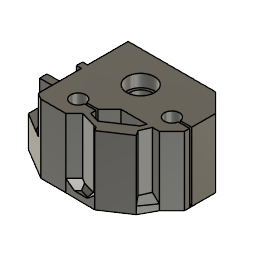
rolls mount right (Autodesk Fusion 360 design; units mm, degrees)
Autodesk Fusion 360 part; units mm, degrees
sketch "Szkic1" plane through (0, 0, 0) normal (0, 0, 1) x (1, 0, 0)
  line L0 (25, -25) -> (25, 25)
  line L1 (35, -10.8) -> (50, -10.8)
  line L2 (35, -9.2) -> (50, -9.2)
  line L3 (-30, -50) -> (0, -50)
  line L4 (0, 0) -> (0, 25)
  line L5 (22, 22) -> (-22, -22) construction
  line L6 (-35.000001, 12.5) -> (-40.000001, 12.5)
  line L7 (-40.000001, 17.5) -> (-40.000001, 12.5)
  line L8 (-30, -25) -> (-30, -50)
  line L9 (-55.000001, 5) -> (-55.000001, -35.000001)
  circle A0 centre (35, -10) radius 6
  line L10 (-25, 25) -> (-35, 25)
  line L11 (-35, 5) -> (-35, 25)
  circle A1 centre (-45, 15) radius 3
  line L12 (-25, 25) -> (-25, -25)
  line L13 (-15, -35.8) -> (0, -35.8)
  line L14 (-15, -34.2) -> (0, -34.2)
  line L15 (-15.5, -15.5) -> (15.5, 15.5) construction
  line L16 (-55, 25) -> (-55.000001, 5)
  line L17 (25, -25) -> (50, -25)
  line L18 (50, -25) -> (50, 5)
  line L19 (-25, -25) -> (-30, -25)
  line L20 (-35, 5) -> (-55.000001, 5)
  line L21 (50, 5) -> (22, 5)
  line L22 (-22, 22) -> (22, -22) construction
  line L23 (-25, -25) -> (25, -25)
  circle A2 centre (-15, -35) radius 6
  line L24 (-35.000001, 17.5) -> (-40.000001, 17.5)
  line L25 (-55.000001, -35.000001) -> (-30, -35.000001)
  line L26 (15.5, -15.5) -> (-14.262563, 14.262563) construction
  line L27 (0, -50) -> (0, -25)
  line L28 (-35, 25) -> (-55, 25)
  line L29 (25, 25) -> (-25, 25)
  circle A3 centre (0, 0) radius 11.5
  line L30 (-55, 25) -> (-55, 60)
  line L31 (-55, 60) -> (-35, 60)
  line L32 (-35, 60) -> (-35, 25)
  circle A4 centre (-45, 45) radius 3
  line L33 (50, 5) -> (25, 25)
  line L34 (-30, -50) -> (-55.000001, -35.000001)
  line L35 (-25, 25) -> (-25, 60)
  line L36 (-25, 60) -> (-35, 60)
  dimension "d2" = 12
  dimension "d3" = 12
  dimension "d6" = 25
  dimension "d11" = 6
  dimension "d12" = 23
  dimension "d13" = 6
  constraint coincident L4.start L5
  constraint coincident L4.start L22
  constraint perpendicular L0 L17
  constraint perpendicular L12 L19
  constraint perpendicular L8 L19
  constraint perpendicular L3 L8
  constraint midpoint L27.end L23
  constraint perpendicular L23 L27
  constraint coincident L4.start A3.centre
  constraint vertical L4
  constraint vertical L11
  constraint coincident L4.start L15
  constraint coincident L4.start L26
  constraint coincident L15.start L5
  constraint vertical L7
  constraint perpendicular L7 L24
  constraint perpendicular L6 L7
  constraint perpendicular L11 L20
  constraint perpendicular L9 L20
  constraint perpendicular L8 L25
  constraint perpendicular L11 L28
  constraint perpendicular L28 L30
  constraint perpendicular L30 L31
  constraint perpendicular L28 L32
  constraint perpendicular L10 L35
  constraint perpendicular L32 L36
  measures "d2" diameter of A2
  measures "d3" diameter of A0
  measures "d6" distance of L4.start L4.end
  measures "d11" diameter of A1
  measures "d12" diameter of A3
  measures "d13" diameter of A4
extrude "Wyciągnięcie proste1" add sketch "Szkic1" along normal blind 10 contours L0 L12 L23 L29 | L0 L1 L2 A0 L17 L18 L21 | L0 L21 L33 | L3 L8 L13 L14 L19 L23 A2 L27 | L8 L9 L10 L11 L12 L19 L20 L25 | L10 L32 L35 L36 | L8 L25 L34 | L6 L7 L11 L24 picked at (-20.495383, -0.188093) picked at (36.89922, -21.986434) picked at (33.333334, 11.666667) picked at (-15.06036, -46.999089) picked at (-46.666667, -18.333334) picked at (-28.333333, 48.333333) picked at (-38.333334, -40) picked at (-38.333334, 15.833334) makes body 1
extrude "Wyciągnięcie proste2" add sketch "Szkic1" against normal blind 10 separate body contours L6 L7 L11 L16 L20 L24 L28 | L28 L30 L31 L32 | L6 L7 L11 L24 picked at (-45.07473, 7.33613) picked at (-44.92527, 30.669463) picked at (-38.333334, 15.833334) makes body 2
extrude "Wyciągnięcie proste3" add sketch "Szkic1" against normal blind 15 contours L0 L12 L23 L29 | L0 L1 L2 A0 L17 L18 L21 | L0 L21 L33 | L3 L8 L13 L14 L19 L23 A2 L27 | L8 L9 L10 L11 L12 L19 L20 L25 | L10 L32 L35 L36 | L8 L25 L34 picked at (-20.495383, -0.188093) picked at (36.89922, -21.986434) picked at (33.333334, 11.666667) picked at (-15.06036, -46.999089) picked at (-46.666667, -18.333334) picked at (-28.333333, 48.333333) picked at (-38.333334, -40) bodies 1 2
sketch "Szkic2" plane through (0, 0, -15) normal (0, 0, -1) x (1, 0, 0)
  circle A0 centre (0, 0) radius 11.5
  line L0 (50, 9.2) -> (40.946428, 9.2)
  arc A1 (40.946427, 10.8) -> (40.946428, 9.2) centre (35, 10) ccw
  line L1 (40.946427, 10.8) -> (50, 10.8)
  line L2 (50, 10.8) -> (50, 25)
  line L3 (50, 25) -> (0, 25)
  line L4 (0, 25) -> (0, 34.2)
  line L5 (0, 34.2) -> (-9.053573, 34.2)
  arc A2 (-9.053573, 35.8) -> (-9.053573, 34.2) centre (-15, 35) ccw
  line L6 (-9.053573, 35.8) -> (0, 35.8)
  line L7 (0, 35.8) -> (0, 50)
  line L8 (0, 50) -> (-30, 50)
  line L9 (-30, 50) -> (-55.000001, 35.000001)
  line L10 (-55.000001, 35.000001) -> (-55.000001, -5)
  line L11 (-55.000001, -5) -> (-35, -5)
  line L12 (-35, -5) -> (-35, -60)
  line L13 (-35, -60) -> (-25, -60)
  line L14 (-25, -60) -> (-25, -25)
  line L15 (-25, -25) -> (25, -25)
  line L16 (25, -25) -> (50, -5)
  line L17 (50, -5) -> (50, 9.2)
  circle A3 centre (0, 0) radius 9
  dimension "d20" = 18
  constraint coincident A0.centre A3.centre
  measures "d20" diameter of A3
extrude "Wyciągnięcie proste4" add sketch "Szkic2" against normal blind 15 contours A0 picked at (10.590344, -1.018455) bodies 1
chamfer "Fazowanie1" distance 9.2 angle 45 1 edges at (0, -25, -2.5) on bodies 1
chamfer "Fazowanie2" distance 10 angle 45 1 edges at (0, -50, -2.5) on bodies 1
chamfer "Fazowanie3" distance 10 angle 45 1 edges at (50, -25, -2.5) on bodies 1
chamfer "Fazowanie4" distance 15 angle 45 1 edges at (-25, 25, -2.5) on bodies 1
sketch "Szkic3" plane through (0, 0, 10) normal (0, 0, 1) x (-1, 0, 0)
  line L0 (-40, 25) -> (-50, 15)
  line L1 (-50, 15) -> (-50, 10.8)
  line L2 (-50, 10.8) -> (-40.946427, 10.8)
  arc A0 (-40.946428, 9.2) -> (-40.946427, 10.8) centre (-35, 10) ccw
  line L3 (-40.946428, 9.2) -> (-50, 9.2)
  line L4 (-50, 9.2) -> (-50, -5)
  line L5 (-50, -5) -> (-25, -25)
  line L6 (-25, -25) -> (10, -25)
  line L7 (10, -25) -> (25, -40)
  line L8 (25, -40) -> (25, -60)
  line L9 (25, -60) -> (35, -60)
  line L10 (35, -60) -> (35.000001, -17.5)
  line L11 (35.000001, -17.5) -> (40.000001, -17.5)
  line L12 (40.000001, -17.5) -> (40.000001, -12.5)
  line L13 (40.000001, -12.5) -> (35, -12.5)
  line L14 (35, -12.5) -> (35, -5)
  line L15 (35, -5) -> (55.000001, -5)
  line L16 (55.000001, -5) -> (55.000001, 35.000001)
  line L17 (55.000001, 35.000001) -> (30, 50)
  line L18 (30, 50) -> (10, 50)
  line L19 (10, 50) -> (0, 40)
  line L20 (0, 40) -> (0, 35.8)
  line L21 (0, 35.8) -> (9.053573, 35.8)
  arc A1 (9.053573, 34.2) -> (9.053573, 35.8) centre (15, 35) ccw
  line L22 (9.053573, 34.2) -> (0, 34.2)
  line L23 (0, 34.2) -> (-9.2, 25)
  line L24 (-9.2, 25) -> (-40, 25)
  circle A2 centre (0, 0) radius 11.5
  line L25 (55.000001, -5) -> (35, -5)
  line L26 (35, -5) -> (35, 5)
  line L27 (35, 5) -> (55.000001, 5)
  line L28 (55.000001, 5) -> (55.000001, -5)
  constraint perpendicular L25 L26
  constraint parallel L25 L27
  constraint parallel L26 L28
  constraint coincident L14.end L15.start
  constraint perpendicular L14 L25
extrude "Wyciągnięcie proste5" add sketch "Szkic3" along normal blind 25 contours L15 L16 L25 L26 L27 L28 picked at (41.666667, 1.666667) bodies 1
sketch "Szkic4" plane through (0, -5, 0) normal (0, -1, 0) x (1, 0, 0)
  line L0 (-55.000001, 10) -> (-35, 10)
  line L1 (-35, 10) -> (-35, 35)
  line L2 (-35, 35) -> (-55.000001, 35)
  line L3 (-55.000001, 35) -> (-55.000001, 10)
  circle A0 centre (-45, 25) radius 3
  dimension "d29" = 6
  measures "d29" diameter of A0
extrude "Wyciągnięcie proste6" cut sketch "Szkic4" against normal blind 32 contours A0 picked at (-45.440071, 26.928078) bodies 1
chamfer "Fazowanie5" distance 5 angle 45 1 edges at (-45, -5, 10) on bodies 1
sketch "Szkic5" plane through (0, -5, 0) normal (0, -1, 0) x (1, 0, 0)
  line L0 (-55.000001, 15) -> (-35, 15)
  line L1 (-35, 15) -> (-35, 35)
  line L2 (-35, 35) -> (-55.000001, 35)
  line L3 (-55.000001, 35) -> (-55.000001, 15)
  circle A0 centre (-45, 25) radius 3
  line L4 (-46.500001, 28) -> (-43.500001, 28)
  line L5 (-43.500001, 28) -> (-43.500001, 26)
  line L6 (-46.500001, 28) -> (-46.500001, 27.795438)
  line L7 (-46.500001, 27.795438) -> (-46.500001, 26)
  constraint horizontal L4
  constraint perpendicular L4 L5
  constraint perpendicular L4 L6
  constraint parallel L6 L7
extrude "Wyciągnięcie proste7" cut sketch "Szkic5" against normal blind 23 contours A0 L4 L5 | A0 L4 L6 L7 picked at (-43.617317, 27.789905) picked at (-46.141503, 27.889805) bodies 1
sketch "Szkic6" plane through (0, 0, -15) normal (0, 0, -1) x (1, 0, 0)
  circle A0 centre (0, 0) radius 9
  line L0 (50, 15) -> (40, 25)
  line L1 (40, 25) -> (9.2, 25)
  line L2 (9.2, 25) -> (0, 34.2)
  line L3 (0, 34.2) -> (-9.053573, 34.2)
  arc A1 (-9.053573, 35.8) -> (-9.053573, 34.2) centre (-15, 35) ccw
  line L4 (-9.053573, 35.8) -> (0, 35.8)
  line L5 (0, 35.8) -> (0, 40)
  line L6 (0, 40) -> (-10, 50)
  line L7 (-10, 50) -> (-30, 50)
  line L8 (-30, 50) -> (-55.000001, 35.000001)
  line L9 (-55.000001, 35.000001) -> (-55.000001, -5)
  line L10 (-55.000001, -5) -> (-35, -5)
  line L11 (-35, -5) -> (-35, -60)
  line L12 (-35, -60) -> (-25, -60)
  line L13 (-25, -60) -> (-25, -40)
  line L14 (-25, -40) -> (-10, -25)
  line L15 (-10, -25) -> (25, -25)
  line L16 (25, -25) -> (50, -5)
  line L17 (50, -5) -> (50, 9.2)
  line L18 (50, 9.2) -> (40.946428, 9.2)
  arc A2 (40.946427, 10.8) -> (40.946428, 9.2) centre (35, 10) ccw
  line L19 (40.946427, 10.8) -> (50, 10.8)
  line L20 (50, 10.8) -> (50, 15)
  line L21 (50, 9.2) -> (40.946428, 9.2)
  line L22 (40.946428, 9.2) -> (40.946427, 10.8)
  line L23 (40.946427, 10.8) -> (50, 10.8)
  line L24 (50, 10.8) -> (50, 9.2)
  line L25 (0, 35.8) -> (-9.053573, 35.8)
  line L26 (-9.053573, 35.8) -> (-9.053573, 34.2)
  line L27 (-9.053573, 34.2) -> (0, 34.2)
  line L28 (0, 34.2) -> (0, 35.8)
  constraint perpendicular L21 L22
  constraint parallel L21 L23
  constraint parallel L22 L24
  constraint parallel L18 L21
  constraint coincident L17.end L18.start
  constraint perpendicular L25 L26
  constraint parallel L25 L27
  constraint parallel L26 L28
  constraint perpendicular L5 L25
  constraint coincident L4.end L5.start
extrude "Wyciągnięcie proste8" add sketch "Szkic6" against normal blind 1 contours L18 L19 L21 L22 L23 L24 | L3 L4 L25 L26 L27 L28 picked at (46.982142, 10.266667) picked at (-3.017858, 34.733333) bodies 1
sketch "Szkic7" plane through (0, 0, -10) normal (0, 0, -1) x (1, 0, 0)
  circle A0 centre (-45, -45) radius 3
  circle A1 centre (-45, -15) radius 3
  line L0 (-55.000001, -5) -> (-55, -25)
  line L1 (-55, -25) -> (-55, -60)
  line L2 (-55, -60) -> (-35, -60)
  line L3 (-35, -60) -> (-35, -5)
  line L4 (-35, -5) -> (-55.000001, -5)
  circle A2 centre (-45, -15) radius 5.5
  circle A3 centre (-45, -45) radius 5.5
  dimension "d37" = 11
  dimension "d38" = 11
  constraint concentric A1 A2
  constraint concentric A0 A3
  measures "d37" diameter of A2
  measures "d38" diameter of A3
extrude "Wyciągnięcie proste9" add sketch "Szkic7" along normal blind 5 contours L0 L1 L2 L3 L4 picked at (-45.137005, -56.828207) bodies 1
extrude "Wyciągnięcie proste10" add sketch "Szkic7" along normal blind 0.2 contours A0 | A1 | A2 | A3 picked at (-45.57473, -43.136771) picked at (-44.709389, -13.071922) picked at (-40.364979, -15.422286) picked at (-40.35381, -45.273244) bodies 1
sketch "Szkic8" plane through (0, 0, 0) normal (0, 0, 1) x (1, 0, 0)
  circle A0 centre (0, 0) radius 11.1
  circle A1 centre (0, 0) radius 11.5
  dimension "d43" = 22.2
  dimension "d44" = 23
  constraint coincident A0.centre A1.centre
  constraint concentric A0 A1
  measures "d43" diameter of A0
  measures "d44" diameter of A1
extrude "Wyciągnięcie proste11" add sketch "Szkic8" along normal blind 10 contours A1 picked at (11.282526, -1.122785) bodies 1
extrude "Wyciągnięcie proste12" cut 1 faces at (-45.222521, 5, 10.691739) along direction (0, -1, 0) blind 25 on bodies 1 bodies 1
extrude "Wyciągnięcie proste13" cut 1 faces at (-40.000001, 15.833334, 3.333333) along direction (1, 0, 0) blind 5 on bodies 1 bodies 1
sketch "Szkic9" plane through (0, 0, 0) normal (0, 0, 1) x (-1, 0, 0)
  line L0 (35, 20) -> (35, -60)
  line L1 (35, -60) -> (55, -60)
  line L2 (55, -60) -> (55, -25)
  line L3 (55, -25) -> (55.000001, -5)
  line L4 (55.000001, -5) -> (55.000001, 20)
  line L5 (55.000001, 20) -> (35, 20)
  circle A0 centre (45, -45) radius 3
  circle A1 centre (45, -15) radius 3
  circle A2 centre (45.000001, 10) radius 3
  line L6 (35.000001, 7.5) -> (35.000001, 12.5)
  line L7 (35.000001, 12.5) -> (39.000001, 12.5)
  line L8 (39.000001, 12.5) -> (39.000001, 7.5)
  line L9 (39.000001, 7.5) -> (35.000001, 7.5)
  dimension "d51" = 6
  dimension "d52" = 4
  constraint perpendicular L6 L7
  constraint parallel L6 L8
  constraint parallel L7 L9
  measures "d51" diameter of A2
extrude "Wyciągnięcie proste14" add sketch "Szkic9" along normal blind 10 contours L0 L6 L7 L8 L9 picked at (37.666667, 9.166667) bodies 1
extrude "Wyciągnięcie proste15" cut sketch "Szkic9" against normal blind 31 contours A2 picked at (44.425271, 11.863229) bodies 1
sketch "Szkic10" plane through (0, 0, 10) normal (0, 0, 1) x (-1, 0, 0)
  line L0 (35, -60) -> (35.000001, 7.5)
  line L1 (35.000001, 7.5) -> (39.000001, 7.5)
  line L2 (39.000001, 7.5) -> (39.000001, 12.5)
  line L3 (39.000001, 12.5) -> (35.000001, 12.5)
  line L4 (35.000001, 12.5) -> (35, 20)
  line L5 (35, 20) -> (55.000001, 20)
  line L6 (55.000001, 20) -> (55.000001, 35.000001)
  line L7 (55.000001, 35.000001) -> (30, 50)
  line L8 (30, 50) -> (10, 50)
  line L9 (10, 50) -> (0, 40)
  line L10 (0, 40) -> (0, 35.8)
  line L11 (0, 35.8) -> (9.053573, 35.8)
  arc A0 (9.053573, 34.2) -> (9.053573, 35.8) centre (15, 35) ccw
  line L12 (9.053573, 34.2) -> (0, 34.2)
  line L13 (0, 34.2) -> (-9.2, 25)
  line L14 (-9.2, 25) -> (-40, 25)
  line L15 (-40, 25) -> (-50, 15)
  line L16 (-50, 15) -> (-50, 10.8)
  line L17 (-50, 10.8) -> (-40.946427, 10.8)
  arc A1 (-40.946428, 9.2) -> (-40.946427, 10.8) centre (-35, 10) ccw
  line L18 (-40.946428, 9.2) -> (-50, 9.2)
  line L19 (-50, 9.2) -> (-50, -5)
  line L20 (-50, -5) -> (-25, -25)
  line L21 (-25, -25) -> (10, -25)
  line L22 (10, -25) -> (25, -40)
  line L23 (25, -40) -> (25, -60)
  line L24 (25, -60) -> (35, -60)
  circle A2 centre (0, 0) radius 11.1
  line L25 (55.000001, 20) -> (35, 20)
  line L26 (35, 20) -> (35, 26)
  line L27 (35, 26) -> (55.000001, 26)
  line L28 (55.000001, 26) -> (55.000001, 20)
  dimension "d57" = 6
  constraint perpendicular L25 L26
  constraint parallel L25 L27
  constraint parallel L26 L28
  constraint coincident L4.end L5.start
  constraint parallel L5 L25
extrude "Wyciągnięcie proste16" add sketch "Szkic10" along normal blind 20 contours L5 L6 L25 L26 L27 L28 picked at (41.666667, 24) bodies 1
sketch "Szkic11" plane through (0, -26, 0) normal (0, -1, 0) x (1, 0, 0)
  line L0 (-55.000001, 10) -> (-35, 10)
  line L1 (-35, 10) -> (-35, 30)
  line L2 (-35, 30) -> (-55.000001, 30)
  line L3 (-55.000001, 30) -> (-55.000001, 10)
  circle A0 centre (-45.000001, 20) radius 3
  dimension "d60" = 6
  measures "d60" diameter of A0
extrude "Wyciągnięcie proste17" cut sketch "Szkic11" against normal blind 26 contours A0 picked at (-45.440072, 21.928078) bodies 1
chamfer "Fazowanie6" distance 20 angle 45 1 edges at (-35, -23, 10) on bodies 1
chamfer "Fazowanie7" distance 3 angle 45 1 edges at (-35, -26, 10) on bodies 1
sketch "Szkic12" plane through (0, 0, -15) normal (0, 0, -1) x (1, 0, 0)
  circle A0 centre (-45.000001, 10) radius 3
  circle A1 centre (-45, -15) radius 5.5
  circle A2 centre (-45, -45) radius 5.5
  arc A3 (40.946427, 10.8) -> (40.946428, 9.2) centre (35, 10) ccw
  line L0 (40.946427, 10.8) -> (40.946428, 9.2)
  line L1 (50, 9.2) -> (50, 10.8)
  line L2 (50, 10.8) -> (50, 15)
  line L3 (50, 15) -> (40, 25)
  line L4 (40, 25) -> (9.2, 25)
  line L5 (9.2, 25) -> (0, 34.2)
  line L6 (0, 34.2) -> (0, 40)
  line L7 (0, 40) -> (-10, 50)
  line L8 (-10, 50) -> (-30, 50)
  line L9 (-30, 50) -> (-55.000001, 35.000001)
  line L10 (-55.000001, 35.000001) -> (-55.000001, -5)
  line L11 (-55.000001, -5) -> (-55, -25)
  line L12 (-55, -25) -> (-55, -60)
  line L13 (-55, -60) -> (-25, -60)
  line L14 (-25, -60) -> (-25, -40)
  line L15 (-25, -40) -> (-10, -25)
  line L16 (-10, -25) -> (25, -25)
  line L17 (25, -25) -> (50, -5)
  line L18 (50, -5) -> (50, 9.2)
  circle A4 centre (0, 0) radius 9
  line L19 (-9.053573, 35.8) -> (-9.053573, 34.2)
  arc A5 (-9.053573, 35.8) -> (-9.053573, 34.2) centre (-15, 35) ccw
  circle A6 centre (-45.000001, 10) radius 5.5
  dimension "d65" = 11
  constraint concentric A0 A6
  measures "d65" diameter of A6
extrude "Wyciągnięcie proste18" cut sketch "Szkic12" against normal blind 5 contours A6 picked at (-40.36498, 9.577714) bodies 1
extrude "Wyciągnięcie proste19" cut 1 faces at (-45.669792, 43.839886, -10.2) along direction (0, 0, 1) blind 0.2 on bodies 1 bodies 1
extrude "Wyciągnięcie proste20" cut 1 faces at (-43.619823, 11.993504, -10.2) along direction (0, 0, 1) blind 0.2 on bodies 1 bodies 1
extrude "Wyciągnięcie proste21" cut 3 faces at (-40.36498, -9.577714, -10) (-40.364979, 15.422286, -10) (-40.364979, 45.422286, -10) along direction (0, 0, 1) blind 4 on bodies 1 bodies 1
sketch "Szkic13" plane through (0, 0, -6) normal (0, 0, -1) x (1, 0, 0)
  circle A0 centre (-45, -45) radius 3
  circle A1 centre (-45, -45) radius 5.5
  circle A2 centre (-45, -15) radius 5.5
  circle A3 centre (-45, -15) radius 5.5
  circle A4 centre (-45, -45) radius 5.5
  circle A5 centre (-45.000001, 10) radius 5.5
  dimension "d75" = 11
  dimension "d76" = 11
  dimension "d77" = 11
  constraint concentric A2 A3
  constraint concentric A0 A4
  measures "d75" diameter of A2
  measures "d76" diameter of A4
  measures "d77" diameter of A5
extrude "Wyciągnięcie proste22" add sketch "Szkic13" 1 faces at (-40.364979, 45.422286, -6) along normal blind 0.2 contours A0 | A2 A3 | A5 picked at (-45.57473, -43.136771) picked at (-43.619823, -11.993504) picked at (-43.856936, 12.514127) on bodies 1 bodies 1
delete_face "Usuń powierzchnię1" 1 faces at (-29.336, -28, 11) on bodies 1
sketch "Szkic14" plane through (0, -26, 0) normal (0, -1, 0) x (1, 0, 0)
  circle A0 centre (-45.000001, 20) radius 3
  line L0 (-55.000001, 10) -> (-15, 10)
  line L1 (-15, 10) -> (-35, 30)
  line L2 (-35, 30) -> (-55.000001, 30)
  line L3 (-55.000001, 30) -> (-55.000001, 10)
  line L4 (-35, 10) -> (-15, 10)
  line L5 (-15, 10) -> (-15, 30)
  line L6 (-15, 30) -> (-35, 30)
  line L7 (-35, 30) -> (-35, 10)
  constraint perpendicular L4 L5
  constraint parallel L4 L6
  constraint parallel L5 L7
  constraint coincident L0.end L1.start
  constraint parallel L0 L4
  constraint midpoint L0 L4.start
extrude "Wyciągnięcie proste23" cut sketch "Szkic14" against normal blind 9 contours L0 L1 L4 L7 picked at (-28.333333, 16.666667) bodies 1
sketch "Szkic15" plane through (0, 0, 10) normal (0, 0, 1) x (-1, 0, 0)
  line L0 (35, 26) -> (55.000001, 26)
  line L1 (55.000001, 26) -> (55.000001, 35.000001)
  line L2 (55.000001, 35.000001) -> (30, 50)
  line L3 (30, 50) -> (10, 50)
  line L4 (10, 50) -> (0, 40)
  line L5 (0, 40) -> (0, 35.8)
  line L6 (0, 35.8) -> (9.053573, 35.8)
  arc A0 (9.053573, 34.2) -> (9.053573, 35.8) centre (15, 35) ccw
  line L7 (9.053573, 34.2) -> (0, 34.2)
  line L8 (0, 34.2) -> (-9.2, 25)
  line L9 (-9.2, 25) -> (-40, 25)
  line L10 (-40, 25) -> (-50, 15)
  line L11 (-50, 15) -> (-50, 10.8)
  line L12 (-50, 10.8) -> (-40.946427, 10.8)
  arc A1 (-40.946428, 9.2) -> (-40.946427, 10.8) centre (-35, 10) ccw
  line L13 (-40.946428, 9.2) -> (-50, 9.2)
  line L14 (-50, 9.2) -> (-50, -5)
  line L15 (-50, -5) -> (-25, -25)
  line L16 (-25, -25) -> (10, -25)
  line L17 (10, -25) -> (25, -40)
  line L18 (25, -40) -> (25, -60)
  line L19 (25, -60) -> (35, -60)
  line L20 (35, -60) -> (35.000001, 7.5)
  line L21 (35.000001, 7.5) -> (39.000001, 7.5)
  line L22 (39.000001, 7.5) -> (39.000001, 12.5)
  line L23 (39.000001, 12.5) -> (35.000001, 12.5)
  line L24 (35.000001, 12.5) -> (35, 20)
  line L25 (35, 20) -> (35, 26)
  circle A2 centre (0, 0) radius 11.1
  line L26 (40.000001, 26) -> (35, 26)
  line L27 (35, 26) -> (35, 47.000001)
  line L28 (40.000001, 26) -> (40.000001, 44.000001)
  line L29 (40.000001, 44.000001) -> (35, 44.000001)
  line L30 (40.000001, 44.000001) -> (35, 47.000001)
  constraint coincident L0.start L25.end
  constraint perpendicular L0 L27
  constraint perpendicular L0 L28
  constraint perpendicular L27 L29
extrude "Wyciągnięcie proste24" add sketch "Szkic15" along normal blind 20 contours L0 L26 L27 L28 L29 picked at (36.666667, 38) bodies 1
chamfer "Fazowanie8" distance 18 angle 45 1 edges at (-37.500001, -44.000001, 30) on bodies 1
chamfer "Fazowanie9" distance 2 angle 45 1 edges at (-37.500001, -44.000001, 10) on bodies 1
extrude "Wyciągnięcie proste25" cut 1 faces at (-40.000001, -32, 17.333333) along direction (1, 0, 0) blind 1 on bodies 1 bodies 1
extrude "Wyciągnięcie proste26" cut 1 faces at (-39.666667, -44.000001, 10.666667) along direction (0, -1, 0) blind 3 on bodies 1 bodies 1
sketch "Szkic16" plane through (0, 0, -15) normal (0, 0, -1) x (1, 0, 0)
  circle A0 centre (-45.000001, 10) radius 5.5
  circle A1 centre (-45, -15) radius 5.5
  circle A2 centre (-45, -45) radius 5.5
  arc A3 (40.946427, 10.8) -> (40.946428, 9.2) centre (35, 10) ccw
  line L0 (40.946427, 10.8) -> (40.946428, 9.2)
  line L1 (50, 9.2) -> (50, 10.8)
  line L2 (50, 10.8) -> (50, 15)
  line L3 (50, 15) -> (40, 25)
  line L4 (40, 25) -> (9.2, 25)
  line L5 (9.2, 25) -> (0, 34.2)
  line L6 (0, 34.2) -> (0, 40)
  line L7 (0, 40) -> (-10, 50)
  line L8 (-10, 50) -> (-30, 50)
  line L9 (-30, 50) -> (-55.000001, 35.000001)
  line L10 (-55.000001, 35.000001) -> (-55.000001, -5)
  line L11 (-55.000001, -5) -> (-55, -25)
  line L12 (-55, -25) -> (-55, -60)
  line L13 (-55, -60) -> (-25, -60)
  line L14 (-25, -60) -> (-25, -40)
  line L15 (-25, -40) -> (-10, -25)
  line L16 (-10, -25) -> (25, -25)
  line L17 (25, -25) -> (50, -5)
  line L18 (50, -5) -> (50, 9.2)
  circle A4 centre (0, 0) radius 9
  line L19 (-9.053573, 35.8) -> (-9.053573, 34.2)
  arc A5 (-9.053573, 35.8) -> (-9.053573, 34.2) centre (-15, 35) ccw
  line L20 (145, 10) -> (65, 10)
  line L21 (145, -20) -> (145, 10)
  line L22 (35, -20) -> (145, -20)
  line L23 (30, -15) -> (35, -20)
  line L24 (-0.000001, -15) -> (30, -15)
  arc A6 (1.994073, -12.846154) -> (-5.238639, 11.897759) centre (0, 0) ccw
  line L25 (-27.009618, 4.292583) -> (-5.238639, 11.897759)
  line L26 (-30, 6.42857) -> (-27.009618, 4.292583)
  line L27 (-30, 20) -> (-30, 6.42857)
  line L28 (-35, 25) -> (-30, 20)
  line L29 (-35, 50) -> (-35, 25)
  line L30 (-25, 60) -> (-35, 50)
  line L31 (-10, 60) -> (-25, 60)
  line L32 (-2.588718, 55.059146) -> (-10, 60)
  line L33 (10.751366, 46.165756) -> (-1.257438, 54.171625)
  line L34 (-1.257438, 54.171625) -> (-8.526939, 43.267374)
  line L35 (-9.858219, 44.154894) -> (-2.588718, 55.059146)
  arc A7 (-9.858219, 44.154894) -> (-8.526939, 43.267374) centre (-15.000002, 35) ccw
  line L36 (25.728271, 30.772825) -> (10.751366, 40.757429)
  line L37 (43.565129, 24.289914) -> (31.062354, 32.625097)
  line L38 (65, 10) -> (44.896409, 23.402394)
  line L39 (44.896409, 23.402394) -> (41.473063, 18.267373)
  line L40 (40.141782, 19.154894) -> (43.565129, 24.289914)
  arc A8 (40.141782, 19.154894) -> (41.473063, 18.267373) centre (35, 10) ccw
  line L41 (30.997923, 38.677303) -> (16.021018, 48.661907)
  line L42 (25.728271, 30.772825) -> (28.224422, 29.108725)
  line L43 (28.224422, 29.108725) -> (33.494074, 37.013203)
  line L44 (33.494074, 37.013203) -> (30.997923, 38.677303)
  line L45 (10.751366, 40.757429) -> (8.255215, 42.42153)
  line L46 (8.255215, 42.42153) -> (13.524867, 50.326007)
  line L47 (13.524867, 50.326007) -> (16.021018, 48.661907)
  line L48 (8.255215, 42.42153) -> (0, 40)
  line L49 (28.224422, 29.108725) -> (30, 25)
  line L50 (7.129321, 46.259806) -> (-1.125894, 43.838276)
  line L51 (31.896231, 30.69549) -> (33.671809, 26.586766)
  line L52 (31.896231, 30.69549) -> (35.227355, 22.987198)
  line L53 (35.227355, 22.987198) -> (34.633269, 24.361926)
  line L54 (33.671809, 26.586766) -> (33.561793, 26.841344)
  line L55 (33.561793, 26.841344) -> (30.056152, 34.95347)
  line L56 (2.347034, 44.857002) -> (9.89339, 47.070599)
  line L57 (4.832074, 45.585947) -> (-3.944934, 43.011358)
  dimension "d91" = 3
  dimension "d92" = 3
  dimension "d93" = 4
  dimension "d94" = -4
  constraint parallel L42 L44
  constraint parallel L45 L47
  constraint coincident L6.end L7.start
  constraint coincident L4 L49.end
  constraint parallel L51 L52
  constraint parallel L52 L55
  constraint parallel L50 L56
  constraint parallel L50 L57
extrude "Wyciągnięcie proste27" add sketch "Szkic16" against normal blind 25 contours L4 L43 L49 L51 L52 L54 L55 | L36 L41 L42 L43 L44 L45 L46 L47 | L7 L33 L46 L48 L50 L56 L57 picked at (30.595405, 26.983356) picked at (17.500218, 40.064054) picked at (3.534083, 42.426177) bodies 1
chamfer "Fazowanie10" distance 1.447778 angle 45 1 edges at (10.751366, -46.165756, -2.5) on bodies 1
sketch "Szkic17" plane through (0, 0, -15) normal (0, 0, -1) x (1, 0, 0)
  line L0 (-3.223097, 43.223097) -> (-10, 50)
  line L1 (-10, 50) -> (-30, 50)
  line L2 (-30, 50) -> (-55.000001, 35.000001)
  line L3 (-55.000001, 35.000001) -> (-55.000001, -5)
  line L4 (-55.000001, -5) -> (-55, -25)
  line L5 (-55, -25) -> (-55, -60)
  line L6 (-55, -60) -> (-25, -60)
  line L7 (-25, -60) -> (-25, -40)
  line L8 (-25, -40) -> (-10, -25)
  line L9 (-10, -25) -> (25, -25)
  line L10 (25, -25) -> (50, -5)
  line L11 (50, -5) -> (50, 9.2)
  line L12 (50, 9.2) -> (50, 10.8)
  line L13 (50, 10.8) -> (50, 15)
  line L14 (50, 15) -> (40, 25)
  line L15 (40, 25) -> (34.357527, 25)
  line L16 (34.357527, 25) -> (30.868196, 33.074385)
  line L17 (30.868196, 33.074385) -> (33.494074, 37.013203)
  line L18 (33.494074, 37.013203) -> (13.524867, 50.326007)
  line L19 (13.524867, 50.326007) -> (11.554449, 47.37038)
  line L20 (11.554449, 47.37038) -> (9.546742, 46.968839)
  line L21 (9.546742, 46.968839) -> (9.546662, 46.968892)
  line L22 (9.546662, 46.968892) -> (-3.223097, 43.223097)
  circle A0 centre (-45.000001, 10) radius 5.5
  circle A1 centre (-45, -15) radius 5.5
  circle A2 centre (-45, -45) radius 5.5
  arc A3 (40.946427, 10.8) -> (40.946428, 9.2) centre (35, 10) ccw
  line L23 (40.946427, 10.8) -> (40.946428, 9.2)
  line L24 (0, 40) -> (8.255215, 42.42153)
  line L25 (8.255215, 42.42153) -> (28.224422, 29.108725)
  line L26 (28.224422, 29.108725) -> (30, 25)
  line L27 (30, 25) -> (9.2, 25)
  line L28 (9.2, 25) -> (0, 34.2)
  line L29 (0, 34.2) -> (0, 40)
  circle A4 centre (0, 0) radius 9
  line L30 (-9.053573, 35.8) -> (-9.053573, 34.2)
  arc A5 (-9.053573, 35.8) -> (-9.053573, 34.2) centre (-15, 35) ccw
  line L31 (40, 25) -> (33.494074, 37.013203)
  line L32 (13.524867, 50.326007) -> (13.080853, 49.659986)
  line L33 (-10, 50) -> (13.524867, 50.326007)
  constraint coincident L14.end L15.start
  constraint coincident L0.end L1.start
extrude "Wyciągnięcie proste28" add sketch "Szkic17" against normal blind 5 contours L0 L19 L20 L22 L32 L33 | L15 L16 L17 L31 picked at (-1.225451, 46.730645) picked at (34.787423, 31.695863) bodies 1
chamfer "Fazowanie11" distance 5 angle 45 1 edges at (32.612861, -29.037192, -10) on bodies 1
chamfer "Fazowanie12" distance 5 angle 45 1 edges at (12.539658, -48.848194, -10) on bodies 1
chamfer "Fazowanie13" distance 5 angle 45 1 edges at (-6.611548, -46.611548, -10) on bodies 1
chamfer "Fazowanie14" distance 3 angle 45 1 edges at (3.241982, -45.11952, -10) on bodies 1
extrude "Wyciągnięcie proste29" cut 1 faces at (-38.333333, 60, -10) along direction (0, -1, 0) blind 25 on bodies 1 bodies 1
extrude "Wyciągnięcie proste30" cut 1 faces at (-25, 38.333334, 1.666667) along direction (1, 0, 0) blind 20 on bodies 1 bodies 1
sketch "Szkic18" plane through (0, 0, -15) normal (0, 0, -1) x (1, 0, 0)
  line L0 (-55, -35) -> (-20, -35)
  line L1 (-20, -35) -> (-10, -25)
  line L2 (-10, -25) -> (25, -25)
  line L3 (25, -25) -> (50, -5)
  line L4 (50, -5) -> (50, 9.2)
  line L5 (50, 9.2) -> (50, 10.8)
  line L6 (50, 10.8) -> (50, 15)
  line L7 (50, 15) -> (40, 25)
  line L8 (40, 25) -> (33.494074, 37.013203)
  line L9 (33.494074, 37.013203) -> (13.524867, 50.326007)
  line L10 (13.524867, 50.326007) -> (-10, 50)
  line L11 (-10, 50) -> (-30, 50)
  line L12 (-30, 50) -> (-55.000001, 35.000001)
  line L13 (-55.000001, 35.000001) -> (-55.000001, -5)
  line L14 (-55.000001, -5) -> (-55, -25)
  line L15 (-55, -25) -> (-55, -35)
  circle A0 centre (-45.000001, 10) radius 5.5
  circle A1 centre (-45, -15) radius 5.5
  arc A2 (40.946427, 10.8) -> (40.946428, 9.2) centre (35, 10) ccw
  line L16 (40.946427, 10.8) -> (40.946428, 9.2)
  line L17 (0, 40) -> (8.255215, 42.42153)
  line L18 (8.255215, 42.42153) -> (28.224422, 29.108725)
  line L19 (28.224422, 29.108725) -> (30, 25)
  line L20 (30, 25) -> (9.2, 25)
  line L21 (9.2, 25) -> (0, 34.2)
  line L22 (0, 34.2) -> (0, 40)
  circle A3 centre (0, 0) radius 9
  line L23 (-9.053573, 35.8) -> (-9.053573, 34.2)
  arc A4 (-9.053573, 35.8) -> (-9.053573, 34.2) centre (-15, 35) ccw
  line L24 (4.999999, -12) -> (39, -12)
  line L25 (39, -12) -> (80, -12)
  line L26 (100, -12) -> (175, -12)
  arc A5 (40.141782, 19.154894) -> (41.473063, 18.267373) centre (35, 10) ccw
  arc A6 (-9.858219, 44.154894) -> (-8.526939, 43.267374) centre (-15.000002, 35) ccw
  line L27 (-24.981369, 11.981369) -> (-18.391605, 7.303082)
  line L28 (-18.391605, 7.303082) -> (-5.238639, 11.897759)
  arc A7 (4.999999, -12) -> (-5.238639, 11.897759) centre (0, 0) ccw
  line L29 (-25, 15) -> (-25, 12)
  line L30 (-35, 25) -> (-25, 15)
  line L31 (-35, 50) -> (-35, 25)
  line L32 (-25, 60) -> (-35, 50)
  line L33 (-9.858219, 44.154894) -> (-2.588718, 55.059146)
  line L34 (-2.588718, 55.059146) -> (-10, 60)
  line L35 (-1.257438, 54.171625) -> (-8.526939, 43.267374)
  line L36 (13.247517, 44.501655) -> (-1.257438, 54.171625)
  line L37 (-35, 25) -> (-35, -11.673177)
  line L38 (-35, -11.673177) -> (4.999999, -12)
  line L39 (35, 10) -> (35, -40)
  line L40 (-55, -35) -> (-35, -35)
  line L41 (-10, -25) -> (-35, -25)
  line L42 (-35, -25) -> (-35, -35)
  constraint parallel L31 L37
  constraint coincident A2.centre A5.centre
  constraint vertical L39
  constraint coincident L0.start L15.end
  constraint coincident L0 L40.end
  constraint coincident L1.end L2.start
  constraint parallel L2 L41
  constraint perpendicular L40 L42
extrude "Wyciągnięcie proste31" cut sketch "Szkic18" against normal blind 40 contours L0 L1 L41 L42 picked at (-21.666667, -28.333334) bodies 1
sketch "Szkic19" plane through (0, 25, 0) normal (0, 1, 0) x (-1, 0, 0)
  line L0 (35, 10) -> (-25, 10)
  line L1 (-25, 10) -> (-25, -15)
  line L2 (-25, -15) -> (35, -15)
  line L3 (35, -15) -> (35, 0)
  line L4 (35, 0) -> (35, 10)
  circle A0 centre (15, -5) radius 2
  circle A1 centre (-20, -5) radius 2
  circle A2 centre (-20, 15) radius 2
  circle A3 centre (15, 15) radius 2
  dimension "d110" = 4
  dimension "d111" = 4
  dimension "d112" = 4
  dimension "d113" = 4
  measures "d110" diameter of A0
  measures "d111" diameter of A1
  measures "d112" diameter of A2
  measures "d113" diameter of A3
extrude "Wyciągnięcie proste32" add 1 faces at (-26.868953, 6.923928, 10) along direction (0, 0, 1) blind 15 on bodies 1 bodies 1
extrude "Wyciągnięcie proste33" cut sketch "Szkic19" against normal blind 10 contours A0 | A1 | A2 | A3 picked at (14.873825, -5.945817) picked at (-20.614877, -5.099362) picked at (-20.614877, 14.900638) picked at (14.606512, 14.182914) bodies 1
delete_face "Usuń powierzchnię2" 1 faces at (41.666667, 11.666667, -1.666667) on bodies 1
chamfer "Fazowanie15" distance 15 distance2 15 1 edges at (50, 25, 5) measured on face at (40.600646, 25, 1.955922) on bodies 1
extrude "Wyciągnięcie proste34" add 1 faces at (10.325167, -0.998583, 0) along direction (0, 0, 1) blind 15 on bodies 1 bodies 1
extrude "Wyciągnięcie proste35" add 1 faces at (-26.868953, 6.923928, 25) along direction (0, 0, 1) blind 15 on bodies 1 bodies 1
extrude "Wyciągnięcie proste36" add 1 faces at (10.325167, -0.998583, 15) along direction (0, 0, 1) blind 15 on bodies 1 bodies 1
extrude "Wyciągnięcie proste37" cut 1 faces at (-35.555556, -46.000001, 30) along direction (0, -1, 0) blind 7 on bodies 1 bodies 1
